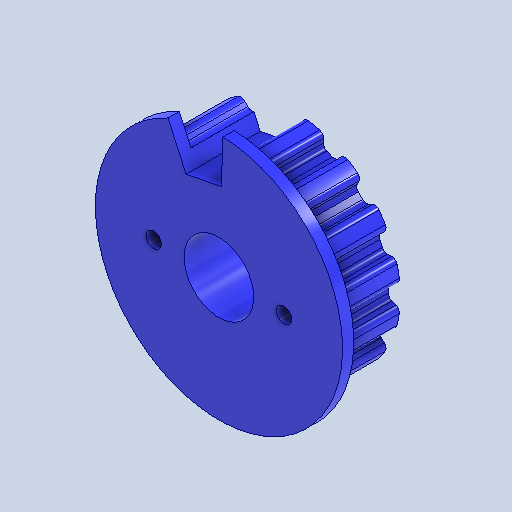
# Autodesk Inventor part: belt_liner_v2_3DP_P-2
Saved by Autodesk Inventor 2025.2 (Build 292293000, 293)
## iProperties
CustomPartVersion: 1
Created: 2024-12-08
Part Number: belt_liner_v2_3DP_P-2
Material: ABS プラスチック
Document SubType Name: Modeling
Designer: haruy
Density: 1.06 g/cm^3
Appearance: 青 - 壁塗料 - 光沢
Author: haruy
Autodesk Inventor part; units mm, degrees
ref_plane "YZ Plane" through (0, 0, 0) normal (1, 0, 0) x (0, 1, 0)
ref_plane "XZ Plane" through (0, 0, 0) normal (0, 1, 0) x (-1, 0, 0)
sketch "プーリ スケッチ" plane through (0, 0, 0) normal (0, 0, 1) x (1, 0, 0)
  circle A0 centre (0, 0) radius 24.2552 construction
  circle A1 centre (0, 0) radius 23.8742
  circle A2 centre (0, 0) radius 21.2072
  line L0 (-2.4489, 23.7483) -> (-1.524, 21.2072)
  line L1 (-1.524, 21.2072) -> (1.524, 21.2072)
  line L2 (1.524, 21.2072) -> (2.4489, 23.7483)
  line L3 (0, 0) -> (0, 23.8742) construction
  point P0 (0, 21.2072)
  dimension "d0" = 48.5104
  dimension "d1" = 0.381
  dimension "d2" = 2.667
  dimension "d3" = 40
  dimension "d4" = 3.048
  constraints: 8 end point, 3 coincident, 3 point on circle, 2 centre point, 1 horizontal, 1 midpoint, 1 point on line, 1 vertical, 1 vertical alignment, 3 other
  measures "d0" diameter of A0
  measures "d1" radial gap between concentric circles of A0 A1
  measures "d3" angle of L2 L0
  measures "d4" distance of L0.end L1.end
extrude "基本ボディ" add sketch "プーリ スケッチ" along normal mid plane 14 contours A2 | A1 L0 L1 L2 | L2 L1 L0 A1
extrude "歯" cut sketch "プーリ スケッチ" along normal through all both and the other way through all contours L2 L1 L0 A1 picked at (0, 22.9759)
fillet "Fillet" radius 1.1938 2 edges at (1.524, 21.2072, 0) (-1.524, 21.2072, 0)
fillet "Fillet" radius 1.1684 4 edges at (-2.4489, 23.7483, 3.5) (-2.4489, 23.7483, -3.5) (2.4489, 23.7483, 3.5) (2.4489, 23.7483, -3.5)
pattern_circular "Teeth" count 16 over 360 about axis through (0, 0, -10) along (0, 0, 1) of "歯", "Fillet"
sketch "スケッチ2" plane through (0, 0, 7) normal (0, 0, 1) x (1, 0, 0)
  circle A0 centre (0, 0) radius 27.5
  dimension "d17" = 55
  constraints: 1 centre point, 1 coincident
  measures "d17" diameter of A0
extrude "押し出し3" add sketch "スケッチ2" along normal blind 2.5
ref_plane "作業平面1" through (0, 0, 0) normal (0, 0, -1) x (-1, 0, 0)
mirror "ミラー1" [suppressed]
sketch "スケッチ3" plane through (0, 0, 9.5) normal (0, 0, 1) x (1, 0, 0)
  circle A0 centre (0, 0) radius 7.75
  circle A1 centre (-9, 0) radius 1.7
  circle A2 centre (9, 0) radius 1.7
  point P0 (-7.6762, 1.0666)
  point P1 (-7.6762, -1.0666)
  point P2 (7.6762, 1.0666)
  point P3 (7.6762, -1.0666)
  dimension "d21" = 15.5
  dimension "d22" = 3.4
  dimension "d23" = 9
  dimension "d26" = 360
  constraints: 3 centre point, 1 coincident, 5 other
  measures "d21" diameter of A0
  measures "d22" diameter of A1
  measures "d23" distance of A1.centre point (0, 0)
extrude "押し出し4" cut sketch "スケッチ3" against normal through all contours A0 A2 | A2 A0 A1 | A1 A0 picked at (7.4644, -0.127) picked at (-7.5945, 0)
sketch "スケッチ4" plane through (0, 0, -7) normal (0, 0, -1) x (-1, 0, 0)
  arc A0 (5.9069, 23.132) -> (3.395, 23.6316) centre (0, 0) ccw projected
  line L0 (3.395, 23.6316) -> (5.9069, 23.132)
  line L1 (4.6509, 23.3818) -> (0, 0)
  line L2 (-6.7344, 25.6465) -> (20.9402, 20.1416)
  line L3 (2.6894, 23.772) -> (6.6125, 22.9916)
  line L4 (6.6125, 22.9916) -> (6.0272, 20.0492)
  line L5 (6.0272, 20.0492) -> (2.1041, 20.8296)
  line L6 (2.1041, 20.8296) -> (2.6894, 23.772)
  line L7 (2.199, 23.8695) -> (7.1029, 22.894)
  line L8 (7.1029, 22.894) -> (9.0538, 32.7019)
  line L9 (9.0538, 32.7019) -> (4.1499, 33.6773)
  line L10 (4.1499, 33.6773) -> (2.199, 23.8695)
  line L11 (-0.1528, 22.2981) -> (8.6743, 20.5423)
  line L12 (8.6743, 20.5423) -> (11.4055, 34.2733)
  line L13 (11.4055, 34.2733) -> (2.5785, 36.0291)
  line L14 (2.5785, 36.0291) -> (-0.1528, 22.2981)
  line L15 (1.118, 26.1237) -> (8.9642, 24.563)
  line L16 (8.9642, 24.563) -> (7.5986, 17.6975)
  line L17 (7.5986, 17.6975) -> (-0.2477, 19.2582)
  line L18 (-0.2477, 19.2582) -> (1.118, 26.1237)
  line L19 (-11.4055, 34.2733) -> (-8.6743, 20.5423)
  line L20 (0.1528, 22.2981) -> (-2.5785, 36.0291)
  line L21 (-7.5986, 17.6975) -> (-8.9642, 24.563)
  line L22 (-1.118, 26.1237) -> (0.2477, 19.2582)
  line L23 (0.2477, 19.2582) -> (-7.5986, 17.6975)
  line L24 (-23.6532, 27.2997) -> (-15.8752, 15.6591)
  line L25 (-8.392, 20.6592) -> (-16.1699, 32.2998)
  line L26 (-13.7927, 13.4425) -> (-17.6817, 19.2628)
  line L27 (-11.03, 23.7073) -> (-7.141, 17.887)
  line L28 (-7.141, 17.887) -> (-13.7927, 13.4425)
  line L29 (-32.2998, 16.1699) -> (-20.6592, 8.392)
  line L30 (-15.6591, 15.8752) -> (-27.2997, 23.6532)
  line L31 (-17.887, 7.141) -> (-23.7073, 11.03)
  line L32 (-19.2628, 17.6817) -> (-13.4425, 13.7927)
  line L33 (-13.4425, 13.7927) -> (-17.887, 7.141)
  line L34 (-36.0291, 2.5785) -> (-22.2981, -0.1528)
  line L35 (-20.5423, 8.6743) -> (-34.2733, 11.4055)
  line L36 (-19.2582, -0.2477) -> (-26.1237, 1.118)
  line L37 (-24.563, 8.9642) -> (-17.6975, 7.5986)
  line L38 (-17.6975, 7.5986) -> (-19.2582, -0.2477)
  line L39 (-34.2733, -11.4055) -> (-20.5423, -8.6743)
  line L40 (-22.2981, 0.1528) -> (-36.0291, -2.5785)
  line L41 (-17.6975, -7.5986) -> (-24.563, -8.9642)
  line L42 (-26.1237, -1.118) -> (-19.2582, 0.2477)
  line L43 (-19.2582, 0.2477) -> (-17.6975, -7.5986)
  line L44 (-27.2997, -23.6532) -> (-15.6591, -15.8752)
  line L45 (-20.6592, -8.392) -> (-32.2998, -16.1699)
  line L46 (-13.4425, -13.7927) -> (-19.2628, -17.6817)
  line L47 (-23.7073, -11.03) -> (-17.887, -7.141)
  line L48 (-17.887, -7.141) -> (-13.4425, -13.7927)
  line L49 (-16.1699, -32.2998) -> (-8.392, -20.6592)
  line L50 (-15.8752, -15.6591) -> (-23.6532, -27.2997)
  line L51 (-7.141, -17.887) -> (-11.03, -23.7073)
  line L52 (-17.6817, -19.2628) -> (-13.7927, -13.4425)
  line L53 (-13.7927, -13.4425) -> (-7.141, -17.887)
  line L54 (-2.5785, -36.0291) -> (0.1528, -22.2981)
  line L55 (-8.6743, -20.5423) -> (-11.4055, -34.2733)
  line L56 (0.2477, -19.2582) -> (-1.118, -26.1237)
  line L57 (-8.9642, -24.563) -> (-7.5986, -17.6975)
  line L58 (-7.5986, -17.6975) -> (0.2477, -19.2582)
  line L59 (11.4055, -34.2733) -> (8.6743, -20.5423)
  line L60 (-0.1528, -22.2981) -> (2.5785, -36.0291)
  line L61 (7.5986, -17.6975) -> (8.9642, -24.563)
  line L62 (1.118, -26.1237) -> (-0.2477, -19.2582)
  line L63 (-0.2477, -19.2582) -> (7.5986, -17.6975)
  line L64 (23.6532, -27.2997) -> (15.8752, -15.6591)
  line L65 (8.392, -20.6592) -> (16.1699, -32.2998)
  line L66 (13.7927, -13.4425) -> (17.6817, -19.2628)
  line L67 (11.03, -23.7073) -> (7.141, -17.887)
  line L68 (7.141, -17.887) -> (13.7927, -13.4425)
  line L69 (32.2998, -16.1699) -> (20.6592, -8.392)
  line L70 (15.6591, -15.8752) -> (27.2997, -23.6532)
  line L71 (17.887, -7.141) -> (23.7073, -11.03)
  line L72 (19.2628, -17.6817) -> (13.4425, -13.7927)
  line L73 (13.4425, -13.7927) -> (17.887, -7.141)
  line L74 (36.0291, -2.5785) -> (22.2981, 0.1528)
  line L75 (20.5423, -8.6743) -> (34.2733, -11.4055)
  line L76 (19.2582, 0.2477) -> (26.1237, -1.118)
  line L77 (24.563, -8.9642) -> (17.6975, -7.5986)
  line L78 (17.6975, -7.5986) -> (19.2582, 0.2477)
  line L79 (34.2733, 11.4055) -> (20.5423, 8.6743)
  line L80 (22.2981, -0.1528) -> (36.0291, 2.5785)
  line L81 (17.6975, 7.5986) -> (24.563, 8.9642)
  line L82 (26.1237, 1.118) -> (19.2582, -0.2477)
  line L83 (19.2582, -0.2477) -> (17.6975, 7.5986)
  line L84 (27.2997, 23.6532) -> (15.6591, 15.8752)
  line L85 (20.6592, 8.392) -> (32.2998, 16.1699)
  line L86 (13.4425, 13.7927) -> (19.2628, 17.6817)
  line L87 (23.7073, 11.03) -> (17.887, 7.141)
  line L88 (17.887, 7.141) -> (13.4425, 13.7927)
  line L89 (16.1699, 32.2998) -> (8.392, 20.6592)
  line L90 (15.8752, 15.6591) -> (23.6532, 27.2997)
  line L91 (7.141, 17.887) -> (11.03, 23.7073)
  line L92 (17.6817, 19.2628) -> (13.7927, 13.4425)
  line L93 (13.7927, 13.4425) -> (7.141, 17.887)
  circle A1 centre (0, 0) radius 27.5
  line L94 (-0.8791, 27.4859) -> (0.7989, 19.05)
  line L95 (11.3306, 25.0573) -> (6.5521, 17.9057)
  line L96 (0.3376, 22.2006) -> (8.1839, 20.6398)
  line L97 (8.1839, 20.6398) -> (7.306, 16.2263)
  line L98 (7.306, 16.2263) -> (-0.5403, 17.787)
  line L99 (-0.5403, 17.787) -> (0.3376, 22.2006)
  line L100 (-0.5403, 17.787) -> (-0.8791, 27.4859)
  line L101 (7.306, 16.2263) -> (11.3306, 25.0573)
  point P0 (6.5521, 17.9057)
  point P1 (12.2913, 26.495)
  point P2 (11.3306, 25.0573)
  point P3 (0.2549, 21.7848)
  point P4 (8.1012, 20.2241)
  point P5 (7.5986, 17.6975)
  point P6 (7.5986, 17.6975)
  point P7 (-0.2477, 19.2582)
  point P8 (-0.2477, 19.2582)
  point P9 (11.3306, 25.0573)
  point P10 (7.3509, 17.7467)
  point P11 (0, 19.2089)
  point P12 (-7.3509, 17.7467)
  point P13 (-13.5828, 13.5828)
  point P14 (-17.7467, 7.3509)
  point P15 (-19.2089, 0)
  point P16 (-17.7467, -7.3509)
  point P17 (-13.5828, -13.5828)
  point P18 (-7.3509, -17.7467)
  point P19 (0, -19.2089)
  point P20 (7.3509, -17.7467)
  point P21 (13.5828, -13.5828)
  point P22 (17.7467, -7.3509)
  point P23 (19.2089, 0)
  point P24 (17.7467, 7.3509)
  point P25 (13.5828, 13.5828)
  point P26 (-0.2477, 19.2582)
  point P27 (-0.2477, 19.2582)
  dimension "d48" = 55
  dimension "d30" = 0
  dimension "d31" = 3
  dimension "d32" = 2
  dimension "d33" = 2
  dimension "d34" = 10
  dimension "d35" = 5
  dimension "d36" = 2.5
  dimension "d37" = 2
  dimension "d38" = 2
  dimension "d41" = 360
  dimension "d46" = 8
  dimension "d47" = 4
  dimension "d65" = 3.5
  dimension "d66" = 13.251
  constraints: 204 end point, 10 parallel, 7 point on line, 5 perpendicular, 2 collinear, 2 midpoint, 2 symmetric about line, 1 coincident, 218 other
  measures "d30" distance between parallel lines of L2 L0
  measures "d31" distance of L3.end L4.end
  measures "d32" distance between parallel lines of L6 L1
  measures "d33" distance between parallel lines of L4 L1
  measures "d34" distance of L8.end L7.end
  measures "d35" distance between parallel lines of L8 L10
  measures "d36" distance between parallel lines of L1 L10
  measures "d37" distance between parallel lines of L10 L14
  measures "d38" distance between parallel lines of L6 L18
  measures "d46" distance of L97.end L98.end
  measures "d47" distance between parallel lines of L1 L99
  measures "d65" distance between parallel lines of L5 L98
extrude "押し出し5" cut sketch "スケッチ4" along normal through all both and the other way through all contours L0 A0 | L2 L4 L11 L1 L0 | A0 L2 L10 L15 L8 | L0 L1 L11 L6 L2 | L2 L16 L11 L4 | L6 L11 L18 L2 | L11 L4 L5 L1 | L1 L5 L6 L11 | L8 L15 L16 L2 | L11 L16 L95 L17 L1 L5 L4 | L2 L18 L15 L10 | L6 L5 L1 L17 L94 L18 L11 | L16 L15 L8 A1 L12 L2 | L2 L12 L89 L95 L11 L16 | L15 L10 A1 L8 | L11 L95 L16 | L18 L11 L94 L20 L14 L2 | L2 L14 A1 L10 L15 L18 | L18 L94 L11 | L17 L93 L97 L98 L1 | L1 L98 L99 L23 L17 | L12 A1 L89 L2 | L2 L89 L12 | L95 L89 L12 L11 | L11 L12 L89 L2 L101 L91 L16 L95 | L16 L91 L93 L17 L95 | L14 L20 L2 | L2 L20 A1 L14 | L94 L18 L22 L100 L2 L20 L14 L11 | L11 L14 L20 L94 | L94 L17 L23 L22 L18 | L89 L101 L2 | L91 L101 L93 L97 L16 | L16 L17 L93 L91 | L2 L100 L20 | L22 L23 L17 L18 | L18 L99 L23 L100 L22 | L97 L93 L101 | L100 L23 L99 | L17 L97 L93 | L23 L99 L17
sketch "スケッチ6" plane through (0, 0, 9.5) normal (0, 0, 1) x (1, 0, 0)
  circle A0 centre (0, 0) radius 7.5 projected
  circle A1 centre (0, 0) radius 8.25
  circle A2 centre (-14.5, 0) radius 4
  circle A3 centre (14.5, 0) radius 4
  circle A4 centre (-14.5, 0) radius 1.7
  circle A5 centre (14.5, 0) radius 1.7
  circle A6 centre (0, 0) radius 8.5
  dimension "d53" = 16.5
  dimension "d54" = 8
  dimension "d55" = 14.5
  dimension "d58" = 360
  dimension "d60" = 3.4
  dimension "d61" = 3.4
  dimension "d64" = 17
  constraints: 6 centre point, 4 coincident, 5 other
  measures "d53" diameter of A1
  measures "d54" diameter of A2
  measures "d55" distance of point (0, 0) A2.centre
  measures "d60" diameter of A4
  measures "d61" diameter of A5
  measures "d64" diameter of A6
extrude "押し出し7" cut sketch "スケッチ6" against normal through all contours A4 | A5
sketch "スケッチ7" plane through (0, 0, 9.5) normal (0, 0, 1) x (1, 0, 0)
  circle A0 centre (14.5, 0) radius 1.7 projected
  circle A1 centre (-14.5, 0) radius 1.7 projected
  line L0 (-7.306, 16.2263) -> (-11.3306, 25.0573) projected
  arc A2 (-11.3306, 25.0573) -> (0.8791, 27.4859) centre (0, 0) ccw projected
  line L1 (0.5403, 17.787) -> (-7.306, 16.2263) projected
  circle A3 centre (0, 0) radius 7.75 projected
  line L2 (0.8791, 27.4859) -> (0.5403, 17.787) projected
equation "\"d1\" = da_a"
equation "\"d2\" = da_hg"
equation "\"d3\" = 2 * da_fi"
equation "\"d4\" = da_bw"
equation "\"d5\" = da_bf"
equation "\"d7\" = da_bf"
equation "\"d9\" = da_rb"
equation "\"d10\" = da_rt"
equation "\"da_pb\" = 9.525"
equation "\"da_fi\" = 20deg"
equation "\"da_hg\" = 2.667"
equation "\"da_bw\" = 3.048"
equation "\"da_rb\" = 1.1938"
equation "\"da_rt\" = 1.1684"
equation "\"da_a\" = 0.381"
equation "\"da_bf\" = 14"
equation "\"da_wf\" = 1.27"
equation "\"da_hf\" = 1.651"
body "Solid1"
